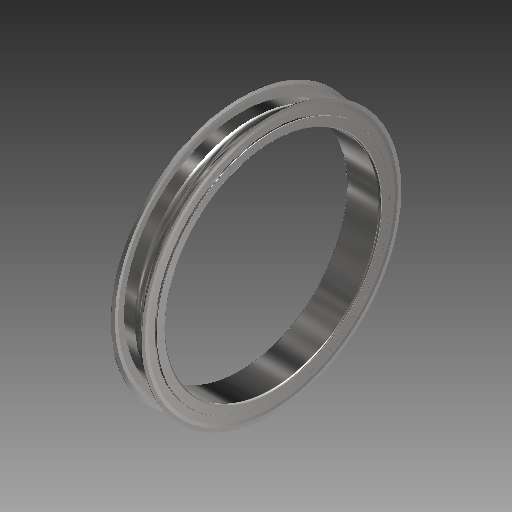
# Autodesk Inventor part: W 61705-2RZ_PART1
Saved by Autodesk Inventor 2018 (Build 220112000, 112)
## iProperties
Category: PARTsolutions
Company: SKF
Part Number: W 61705-2RZ_PART1
Material: Stainless Steel
Catalog Web Link: www.cadenas.de
Description: -Deep groove ball bearings
Vendor: SKF
Document SubType Name: Modeling
Designer: partserver
Manufacturer: SKF
Mass: 3.08279 g
Surface Area: 13.8017 cm^2
Volume: 0.385348 cm^3
Density: 8 g/cm^3
Appearance: Semi-Polished
PSOL_IDENT_0: {$CADENAS_DATA\23d-libs\skf\bearings_units_and_housings\ball_bearings\deep_groove_ball_bearings\bb1_
PSOL_IDENT_1: 001_101.prj},201 {VTYP=3D},{NB=W 61705-2RZ_PART1},{LINA=W 61705-2RZ_PART1},{NN=BB1_001_101_PART1},{N
PSOL_IDENT_2: OPRJ=TRUE},{DATE=19.12.2019 14:34:47},{GEOMDATE=18.12.2019 13:53:11},{VERSION=},{LINEID=17800},{WBVA
PSOL_IDENT_3: R=},{WBNUMERIC=}  {NB=W 61705-2RZ_PART1},{LINA=W 61705-2RZ_PART1},{KT=DUMMY},{PRODUCTID=},{DESIGNATI
PSOL_IDENT_4: ON=W 61705-2RZ},{DD=25.000},{D=32.000},{B=4.000},{C=0.000},{DD1=27.27},{DD2=0.00},{D1=0.00},{D2=30.2
PSOL_IDENT_5: 9},{D3=0.000},{D4=0.000},{HH=MIN},{BB=0.000},{FF=0.00},{R0MAX=MIN},{R0=MIN},{R12=0.20},{PITCH=28.50}
PSOL_IDENT_6: ,{DW=1.588},{DDAMIN=26.500},{DDAMAX=27.000},{DDBMIN=MIN},{DDBMAX=MIN},{DBMIN=MIN},{DAMAX=30.500},{BB
PSOL_IDENT_7: AMIN=MIN},{CAMAX=MIN},{RAMAX=0.200},{LOAD1=0.618},{LOAD2=0.465},{LOAD3=0.020},{SPEED1=43000},{SPEED2=
PSOL_IDENT_8: 20000},{KR=0.015},{F0=8.800},{Z=21},{II=1},{MASS=0.007},{BEARING=W 61705-2RZ},{RING=},{HELP=1.218},{
PSOL_IDENT_9: HELP2=0.855},{DD1ALG=13.635},{YALG=13.635},{PITCH1=28.500},{DW1=1.588},{YALG1=14.782},{HALG1=1.218},
PSOL_IDENT_10: {SH=13.635},{CU=0.482},{DESIGN=dgbb2rs},{HALG=1.135},{B1=0},{SHIELDHELP=2}
NB: W 61705-2RZ_PART1
NT: Deep groove ball bearings
NBSYN: $DESIGNATION._PART1
LINA: W 61705-2RZ_PART1
CATALOG: SKF
SUPPLIER: SKF
ARTICLENO: W 61705-2RZ_PART1
BOMINFO: W 61705-2RZ_PART1
CREATOR: CADENAS GmbH
Title: W 61705-2RZ_PART1
Author: Cadenas PARTsolutions
Comments: Deep groove ball bearings
Autodesk Inventor part; units mm, degrees
ref_plane "YZ Plane" through (0, 0, 0) normal (1, 0, 0) x (0, 1, 0)
ref_plane "XZ Plane" through (0, 0, 0) normal (0, 1, 0) x (-1, 0, 0)
ref_plane "XY Plane" through (0, 0, 0) normal (0, 0, 1) x (1, 0, 0)
sketch "Sketch_58" plane through (0, 0, 0) normal (0, 0, 1) x (1, 0, 0)
  line L0 (50, 0) -> (-50, 0)
  line L1 (0, 13.5683) -> (0, 12.7)
  arc A0 (0, 12.7) -> (0.2, 12.5) centre (0.2, 12.7) ccw
  line L2 (0.2, 12.5) -> (3.8, 12.5)
  arc A1 (3.8, 12.5) -> (4, 12.7) centre (3.8, 12.7) ccw
  line L3 (4, 12.7) -> (4, 13.5683)
  arc A2 (4, 13.5683) -> (3.9333, 13.635) centre (3.9333, 13.5683) ccw
  line L4 (3.9333, 13.635) -> (2.5022, 13.635)
  arc A3 (1.4978, 13.635) -> (2.5022, 13.635) centre (2, 14.25) ccw
  line L5 (1.4978, 13.635) -> (0.0667, 13.635)
  arc A4 (0.0667, 13.635) -> (0, 13.5683) centre (0.0667, 13.5683) ccw
  constraints: 12 end point, 10 point on circle, 5 centre point
revolve "Revolution1" add sketch "Sketch_58" angle 360 about axis through (50, 0, 0) along (1, 0, 0)
sketch "Sketch_60" plane through (0, 0, 0) normal (0, 0, 1) x (1, 0, 0)
  line L0 (50, 0) -> (-50, 0)
  line L1 (0.18, 15.145) -> (0.21, 14.7675)
  line L2 (0.21, 14.7675) -> (0.18, 14.39)
  line L3 (0.18, 14.39) -> (0.18, 13.635)
  line L4 (0.18, 13.635) -> (0.24, 13.635)
  line L5 (0.24, 13.635) -> (0.3, 14.39)
  line L6 (0.3, 14.39) -> (0.3, 14.7675)
  line L7 (0.3, 14.7675) -> (0.24, 15.145)
  line L8 (0.24, 15.145) -> (0.18, 15.145)
  constraints: 18 end point
revolve "Revolution2" add sketch "Sketch_60" angle 360 about axis through (50, 0, 0) along (1, 0, 0)
sketch "Sketch_61" plane through (0, 0, 0) normal (0, 0, 1) x (1, 0, 0)
  line L0 (50, 0) -> (-50, 0)
  line L1 (3.7, 14.39) -> (3.76, 13.635)
  line L2 (3.76, 13.635) -> (3.82, 13.635)
  line L3 (3.82, 13.635) -> (3.82, 14.39)
  line L4 (3.82, 14.39) -> (3.79, 14.7675)
  line L5 (3.79, 14.7675) -> (3.82, 15.145)
  line L6 (3.82, 15.145) -> (3.76, 15.145)
  line L7 (3.76, 15.145) -> (3.7, 14.7675)
  line L8 (3.7, 14.7675) -> (3.7, 14.39)
  constraints: 18 end point
revolve "Revolution3" add sketch "Sketch_61" angle 360 about axis through (50, 0, 0) along (1, 0, 0)
body "Solid1"
